Autodesk Inventor part; units mm, degrees
(part 4 of 4)
body "Solid1"
